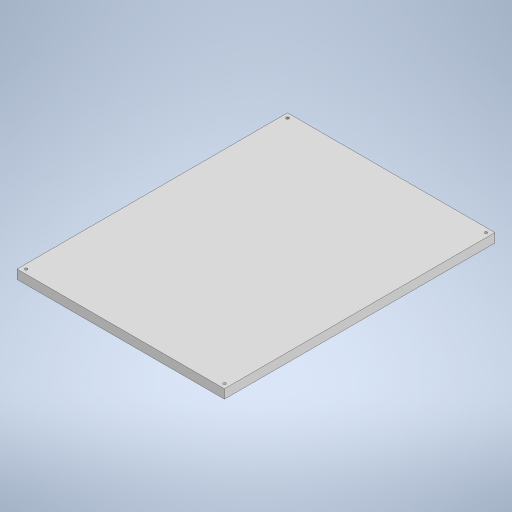
# Autodesk Inventor part: base di lavoro sopra
Saved by Autodesk Inventor 2024 (Build 280153000, 153)
## iProperties
Created: 2024-04-11
Part Number: base di lavoro sopra
Material: Generico
Document SubType Name: Modeling
Designer: Giorgio
Density: 1 g/cm^3
Appearance: Default
Author: Giorgio
Autodesk Inventor part; units mm, degrees
ref_plane "YZ Plane" through (0, 0, 0) normal (1, 0, 0) x (0, 1, 0)
ref_plane "XZ Plane" through (0, 0, 0) normal (0, 1, 0) x (-1, 0, 0)
ref_plane "XY Plane" through (0, 0, 0) normal (0, 0, 1) x (1, 0, 0)
sketch "Schizzo1" plane through (0, 0, 0) normal (0, 1, 0) x (-1, 0, 0)
  line L0 (112.9076, 150.0243) -> (-117.0924, 150.0243)
  line L1 (-117.0924, -149.9757) -> (112.9076, -149.9757)
  line L2 (112.9076, -149.9757) -> (112.9076, 150.0243)
  circle A0 centre (43.9076, 95.0243) radius 2.75
  circle A1 centre (43.9076, 65.0243) radius 2.75
  circle A2 centre (11.9076, 95.0243) radius 2.75
  circle A3 centre (11.9076, 65.0243) radius 2.75
  circle A4 centre (43.9076, -64.9757) radius 2.75
  circle A5 centre (43.9076, -94.9757) radius 2.75
  circle A6 centre (11.9076, -64.9757) radius 2.75
  circle A7 centre (11.9076, -94.9757) radius 2.75
  circle A8 centre (-16.0924, 95.0243) radius 2.75
  circle A9 centre (-16.0924, 65.0243) radius 2.75
  circle A10 centre (-48.0924, 95.0243) radius 2.75
  circle A11 centre (-48.0924, 65.0243) radius 2.75
  circle A12 centre (-16.0924, -64.9757) radius 2.75
  circle A13 centre (-16.0924, -94.9757) radius 2.75
  circle A14 centre (-48.0924, -64.9757) radius 2.75
  circle A15 centre (-48.0924, -94.9757) radius 2.75
  circle A16 centre (7.9076, 140.0243) radius 3
  circle A17 centre (-12.0924, 140.0243) radius 3
  circle A18 centre (107.9076, 145.0243) radius 1.5
  circle A19 centre (107.9076, -144.9757) radius 1.5
  circle A20 centre (-112.0924, 145.0243) radius 1.5
  circle A21 centre (-112.0924, -144.9757) radius 1.5
  line L3 (85.0682, 741.7724) -> (-144.9318, 741.7724)
  line L4 (-144.9318, 741.7724) -> (-144.9318, 441.7724)
  line L5 (-144.9318, 441.7724) -> (85.0682, 441.7724)
  line L6 (85.0682, 441.7724) -> (85.0682, 741.7724)
  circle A22 centre (80.0682, 736.7724) radius 1.5
  circle A23 centre (80.0682, 446.7724) radius 1.5
  circle A24 centre (-139.9318, 736.7724) radius 1.5
  circle A25 centre (-139.9318, 446.7724) radius 1.5
  dimension "d23" = 30
  dimension "d24" = 32
  dimension "d25" = 160
  dimension "d26" = 60
  dimension "d30" = 20
  dimension "d36" = 290
  dimension "d37" = 220
  dimension "d41" = 230
  dimension "d42" = 300
  dimension "d43" = 3
  dimension "d44" = 5
  dimension "d45" = 5
  dimension "d48" = 290
  dimension "d51" = 220
  constraints: 26 centre point, 14 end point, 6 horizontal, 4 vertical, 2 parallel, 1 perpendicular, 44 other
  measures "d23" distance of A0.centre A1.centre
  measures "d24" distance of A0.centre A2.centre
  measures "d25" distance of A0.centre A4.centre
  measures "d26" distance of A0.centre A8.centre
  measures "d30" distance of A16.centre A17.centre
  measures "d36" distance of A18.centre A19.centre
  measures "d37" distance of A18.centre A20.centre
  measures "d41" distance of L4.end L5.end
  measures "d42" distance of L5.end L3.start
  measures "d43" diameter of A22
  measures "d44" distance from line of L3 A22.centre
  measures "d45" distance from line of L6 A22.centre
  measures "d48" distance of A22.centre A23.centre
  measures "d51" distance of A22.centre A24.centre
extrude "Estrusione1" add sketch "Schizzo1" along normal blind 10 contours L6 L5 L4 L3
